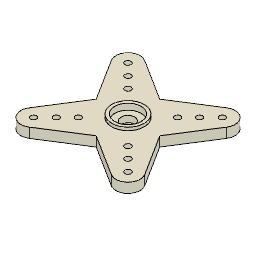
Square Servo Attachment (Autodesk Fusion 360 design; units mm, degrees)
Autodesk Fusion 360 part; units mm, degrees
sketch "Sketch1" plane through (0, 0, 0) normal (0, 1, 0) x (1, 0, 0)
  circle A0 centre (0, 0) radius 3.3909
  circle A1 centre (0, 0) radius 2.3368
  dimension "d1" = 6.7818
  dimension "d2" = 4.6736
  constraint coincident A0.centre A1.centre
  measures "d1" diameter of A0
  measures "d2" diameter of A1
extrude "Extrude1" add sketch "Sketch1" along normal blind 1.9304
sketch "Sketch2" plane through (0, 1.9304, 0) normal (0, 1, 0) x (-1, 0, 0)
  circle A0 centre (0, 0) radius 2.3368
  circle A1 centre (0, 0) radius 3.3909
  line L0 (-10.0076, 10.0076) -> (10.0076, 10.0076) construction
  line L1 (10.0076, 10.0076) -> (10.0076, -10.0076) construction
  line L2 (10.0076, -10.0076) -> (-10.0076, -10.0076) construction
  line L3 (-10.0076, -10.0076) -> (-10.0076, 10.0076) construction
  line L4 (-10.0076, 10.0076) -> (10.0076, -10.0076) construction
  line L5 (10.0076, 10.0076) -> (-10.0076, -10.0076) construction
  circle A2 centre (7.9709, -7.9709) radius 2.0367 construction
  circle A3 centre (-7.9709, -7.9709) radius 2.0367 construction
  circle A4 centre (-7.9709, 7.9709) radius 2.0367 construction
  circle A5 centre (7.9709, 7.9709) radius 2.0367 construction
  circle A6 centre (0, 0) radius 5.334 construction
  circle A7 centre (7.9709, -7.9709) radius 0.5
  circle A8 centre (-7.9709, -7.9709) radius 0.5
  circle A9 centre (7.9709, 7.9709) radius 0.5
  circle A10 centre (-7.9709, 7.9709) radius 0.5
  line L6 (8.4709, -7.9709) -> (-8.4709, -7.9709) construction
  line L7 (0, -5.334) -> (0, 5.334) construction
  line L8 (5.334, 0) -> (-5.334, 0) construction
  line L9 (9.4111, -6.5307) -> (6.5307, -9.4111) construction
  line L10 (-6.5307, -9.4111) -> (-9.4111, -6.5307) construction
  line L11 (-9.4111, 6.5307) -> (-6.5307, 9.4111) construction
  line L12 (9.4111, 6.5307) -> (6.5307, 9.4111) construction
  line L13 (5.334, 0) -> (9.6916, -6.8813)
  line L14 (5.334, 0) -> (9.6916, 6.8813)
  line L15 (0, 5.334) -> (6.8813, 9.6916)
  line L16 (0, 5.334) -> (-6.8813, 9.6916)
  line L17 (-5.334, 0) -> (-9.6916, 6.8813)
  line L18 (-5.334, 0) -> (-9.6916, -6.8813)
  line L19 (0, -5.334) -> (-6.8813, -9.6916)
  line L20 (0, -5.334) -> (6.8813, -9.6916)
  arc A11 (6.8813, -9.6916) -> (9.6916, -6.8813) centre (7.9709, -7.9709) ccw
  arc A12 (-9.6916, -6.8813) -> (-6.8813, -9.6916) centre (-7.9709, -7.9709) ccw
  arc A13 (-6.8813, 9.6916) -> (-9.6916, 6.8813) centre (-7.9709, 7.9709) ccw
  arc A14 (9.6916, 6.8813) -> (6.8813, 9.6916) centre (7.9709, 7.9709) ccw
  circle A15 centre (0, 0) radius 1.143
  dimension "d5" = 20.0152
  dimension "d6" = 20.0152
  dimension "d7" = 10.668
  dimension "d8" = 1
  dimension "d9" = 16.9418
  dimension "d10" = 2.286
  constraint horizontal L0
  constraint perpendicular L0 L1
  constraint parallel L0 L2
  constraint parallel L1 L3
  constraint coincident L4 A0.centre
  constraint coincident L5 A0.centre
  constraint coincident A0.centre A1.centre
  constraint coincident L4 A2.centre
  constraint coincident L5 A3.centre
  constraint coincident L4 A4.centre
  constraint coincident L5 A5.centre
  constraint tangent L2 A2
  constraint tangent L2 A3
  constraint tangent L3 A4
  constraint tangent L0 A5
  constraint equal A2 A3
  constraint equal A2 A4
  constraint equal A2 A5
  constraint concentric A2 A7
  constraint concentric A3 A8
  constraint concentric A5 A9
  constraint concentric A4 A10
  constraint equal A7 A8
  constraint equal A7 A9
  constraint equal A7 A10
  constraint coincident A7 L6.start
  constraint coincident A8 L6.end
  constraint coincident A2.centre L6
  constraint coincident A3.centre L6
  constraint coincident A6 L7.start
  constraint coincident A6 L7.end
  constraint coincident A0.centre L7
  constraint vertical L7
  constraint coincident A6 L8.start
  constraint coincident A6 L8.end
  constraint coincident A0.centre L8
  constraint horizontal L8
  constraint coincident A2 L9.start
  constraint coincident A2 L9.end
  constraint coincident A3 L10.start
  constraint coincident A3 L10.end
  constraint coincident A4 L11.start
  constraint coincident A4 L11.end
  constraint coincident A5 L12.start
  constraint coincident A5 L12.end
  constraint perpendicular L11 L12
  constraint coincident A2.centre L9
  constraint coincident A3.centre L10
  constraint coincident A4.centre L11
  constraint coincident A5.centre L12
  constraint perpendicular L4 L9
  constraint perpendicular L5 L10
  constraint perpendicular L4 L11
  constraint coincident A2 L13.end
  constraint coincident A5 L14.end
  constraint tangent A5 L14
  constraint coincident A5 L15.end
  constraint tangent A5 L15
  constraint coincident A4 L16.end
  constraint coincident A4 L17.end
  constraint tangent A4 L17
  constraint coincident A3 L18.end
  constraint coincident A3 L19.end
  constraint tangent A3 L19
  constraint coincident A2 L20.end
  constraint tangent A2 L13
  constraint tangent A2 L20
  constraint tangent A3 L18
  constraint tangent A4 L16
  constraint tangent L20 A11
  constraint tangent L18 A12
  constraint tangent L16 A13
  constraint tangent L15 A14
  measures "d5" distance of L1.end L2.end
  measures "d6" distance of L0.end L1.end
  measures "d7" diameter of A6
  measures "d8" diameter of A7
  measures "d9" distance of L6.start L6.end
  measures "d10" diameter of A15
extrude "Extrude2" add sketch "Sketch2" along normal blind 1.651 contours A0 | A1 | A7 | A8 | A9 | A10 | L13 L14 L15 L16 L17 L18 L19 L20 A11 A12 A13 A14
sketch "Sketch3" plane through (0, 3.5814, 0) normal (0, 1, 0) x (-1, 0, 0)
  circle A0 centre (0, 0) radius 1.143
  line L0 (5.334, 0) -> (9.6916, 6.8813)
  arc A1 (9.6916, 6.8813) -> (6.8813, 9.6916) centre (7.9709, 7.9709) ccw
  line L1 (6.8813, 9.6916) -> (0, 5.334)
  line L2 (0, 5.334) -> (-6.8813, 9.6916)
  arc A2 (-6.8813, 9.6916) -> (-9.6916, 6.8813) centre (-7.9709, 7.9709) ccw
  line L3 (-9.6916, 6.8813) -> (-5.334, 0)
  line L4 (-5.334, 0) -> (-9.6916, -6.8813)
  arc A3 (-9.6916, -6.8813) -> (-6.8813, -9.6916) centre (-7.9709, -7.9709) ccw
  line L5 (-6.8813, -9.6916) -> (0, -5.334)
  line L6 (0, -5.334) -> (6.8813, -9.6916)
  arc A4 (6.8813, -9.6916) -> (9.6916, -6.8813) centre (7.9709, -7.9709) ccw
  line L7 (9.6916, -6.8813) -> (5.334, 0)
  line L8 (-10.0076, 10.0076) -> (10.0076, 10.0076) construction
  line L9 (10.0076, 10.0076) -> (10.0076, -10.0076) construction
  line L10 (10.0076, -10.0076) -> (-10.0076, -10.0076) construction
  line L11 (-10.0076, -10.0076) -> (-10.0076, 10.0076) construction
  line L12 (-10.0076, 10.0076) -> (10.0076, -10.0076) construction
  line L13 (10.0076, 10.0076) -> (-10.0076, -10.0076) construction
  line L14 (8.2888, -8.2888) -> (-8.2888, 8.2888) construction
  line L15 (-8.2888, -8.2888) -> (8.2888, 8.2888) construction
  line L16 (-8.4455, 8.4455) -> (8.4455, 8.4455) construction
  line L17 (8.4455, 8.4455) -> (8.4455, -8.4455) construction
  line L18 (8.4455, -8.4455) -> (-8.4455, -8.4455) construction
  line L19 (-8.4455, -8.4455) -> (-8.4455, 8.4455) construction
  line L20 (-8.4455, 8.4455) -> (8.4455, -8.4455) construction
  line L21 (8.4455, 8.4455) -> (-8.4455, -8.4455) construction
  circle A5 centre (7.9104, -7.9104) radius 0.5351
  circle A6 centre (-7.9104, -7.9104) radius 0.5351
  circle A7 centre (-7.9104, 7.9104) radius 0.5351
  circle A8 centre (7.9104, 7.9104) radius 0.5351
  line L22 (-6.376, 6.376) -> (6.376, 6.376) construction
  line L23 (6.376, 6.376) -> (6.376, -6.376) construction
  line L24 (6.376, -6.376) -> (-6.376, -6.376) construction
  line L25 (-6.376, -6.376) -> (-6.376, 6.376) construction
  line L26 (-6.376, 6.376) -> (6.376, -6.376) construction
  line L27 (6.376, 6.376) -> (-6.376, -6.376) construction
  line L28 (-6.5278, 6.5278) -> (6.5278, 6.5278) construction
  line L29 (6.5278, 6.5278) -> (6.5278, -6.5278) construction
  line L30 (6.5278, -6.5278) -> (-6.5278, -6.5278) construction
  line L31 (-6.5278, -6.5278) -> (-6.5278, 6.5278) construction
  line L32 (-6.5278, 6.5278) -> (6.5278, -6.5278) construction
  line L33 (6.5278, 6.5278) -> (-6.5278, -6.5278) construction
  circle A9 centre (6.0095, -6.0095) radius 0.5183
  circle A10 centre (-6.0095, -6.0095) radius 0.5183
  circle A11 centre (-6.0095, 6.0095) radius 0.5183
  circle A12 centre (6.0095, 6.0095) radius 0.5183
  line L34 (-4.826, -4.826) -> (4.826, -4.826) construction
  line L35 (4.826, -4.826) -> (4.826, 4.826) construction
  line L36 (4.826, 4.826) -> (-4.826, 4.826) construction
  line L37 (-4.826, 4.826) -> (-4.826, -4.826) construction
  line L38 (-4.826, -4.826) -> (4.826, 4.826) construction
  line L39 (4.826, -4.826) -> (-4.826, 4.826) construction
  line L40 (-4.6338, -4.6338) -> (4.6338, -4.6338) construction
  line L41 (4.6338, -4.6338) -> (4.6338, 4.6338) construction
  line L42 (4.6338, 4.6338) -> (-4.6338, 4.6338) construction
  line L43 (-4.6338, 4.6338) -> (-4.6338, -4.6338) construction
  line L44 (-4.6338, -4.6338) -> (4.6338, 4.6338) construction
  line L45 (4.6338, -4.6338) -> (-4.6338, 4.6338) construction
  circle A13 centre (4.1698, -4.1698) radius 0.6562
  circle A14 centre (-4.1698, -4.1698) radius 0.6562
  circle A15 centre (-4.1698, 4.1698) radius 0.6562
  circle A16 centre (4.1698, 4.1698) radius 0.6562
  dimension "d13" = 23.4442
  dimension "d14" = 16.891
  dimension "d15" = 16.891
  dimension "d16" = 18.034
  dimension "d17" = 13.0556
  dimension "d18" = 13.1064
  dimension "d19" = 9.652
  constraint horizontal L8
  constraint perpendicular L8 L9
  constraint parallel L8 L10
  constraint parallel L9 L11
  constraint coincident L12 A0.centre
  constraint coincident L13 A0.centre
  constraint coincident A0.centre origin
  constraint tangent A4 L10
  constraint tangent A4 L9
  constraint coincident L12 L14.start
  constraint coincident L12 L14.end
  constraint midpoint A0.centre L14
  constraint coincident L13 L15.start
  constraint coincident L13 L15.end
  constraint midpoint A0.centre L15
  constraint equal L14 L15
  constraint horizontal L16
  constraint perpendicular L16 L17
  constraint parallel L16 L18
  constraint parallel L17 L19
  constraint coincident L20 A0.centre
  constraint coincident L21 A0.centre
  constraint coincident L12 A5.centre
  constraint coincident L15 A6.centre
  constraint coincident L14 A7.centre
  constraint coincident L21 A8.centre
  constraint coincident L14.start A5
  constraint coincident L15.start A6
  constraint coincident L14.end A7
  constraint coincident L15.end A8
  constraint tangent L18 A5
  constraint tangent L19 A6
  constraint tangent L19 A7
  constraint tangent L17 A8
  constraint horizontal L22
  constraint perpendicular L22 L23
  constraint parallel L22 L24
  constraint parallel L23 L25
  constraint coincident L26 A0.centre
  constraint coincident L27 A0.centre
  constraint coincident L20 L22.start
  constraint horizontal L28
  constraint perpendicular L28 L29
  constraint parallel L28 L30
  constraint parallel L29 L31
  constraint coincident L32 A0.centre
  constraint coincident L33 A0.centre
  constraint coincident L20 L28.start
  constraint coincident L14 A9.centre
  constraint coincident L33 A10.centre
  constraint coincident L32 A11.centre
  constraint coincident L33 A12.centre
  constraint coincident L23.end A9
  constraint coincident L24.end A10
  constraint coincident L22.start A11
  constraint coincident L22.end A12
  constraint tangent L30 A9
  constraint tangent L30 A10
  constraint tangent L28 A11
  constraint tangent L28 A12
  constraint horizontal L34
  constraint perpendicular L34 L35
  constraint parallel L34 L36
  constraint parallel L35 L37
  constraint coincident L38 A0.centre
  constraint coincident L39 A0.centre
  constraint coincident L15 L34.start
  constraint horizontal L40
  constraint perpendicular L40 L41
  constraint parallel L40 L42
  constraint parallel L41 L43
  constraint coincident L44 A0.centre
  constraint coincident L45 A0.centre
  constraint coincident L21 L40.start
  constraint coincident L39 A13.centre
  constraint coincident L13 A14.centre
  constraint coincident L26 A15.centre
  constraint coincident L15 A16.centre
  constraint coincident L40.end A13
  constraint coincident L40.start A14
  constraint coincident L42.end A15
  constraint coincident L41.end A16
  constraint tangent L34 A13
  constraint tangent L37 A14
  constraint tangent L37 A15
  constraint tangent L36 A16
  measures "d13" distance of L14.start L14.end
  measures "d14" distance of L17.end L18.end
  measures "d15" distance of L16.end L17.end
  measures "d16" distance of L22.start L23.end
  measures "d17" distance of L29.end L30.end
  measures "d18" distance of L40.end L42.end
  measures "d19" distance of L34.start L34.end
hole "Hole1" at (-7.9104, 3.5814, -7.9104) at (-6.0095, 3.5814, -6.0095) at (-4.1698, 3.5814, -4.1698) at (-7.9104, 3.5814, 7.9104) at (-6.0095, 3.5814, 6.0095) at (-4.1698, 3.5814, 4.1698) at (7.9104, 3.5814, 7.9104) at (6.0095, 3.5814, 6.0095) at (4.1698, 3.5814, 4.1698) at (7.9104, 3.5814, -7.9104) at (6.0095, 3.5814, -6.0095) at (4.1698, 3.5814, -4.1698) direction (0, -1, 0) diameter 1 end through all
sketch "Sketch4" plane through (0, 3.5814, 0) normal (0, 1, 0) x (-1, 0, 0)
  circle A0 centre (-6.0095, -6.0095) radius 0.5
  circle A1 centre (-4.1698, 4.1698) radius 0.5
  circle A2 centre (-7.9104, 7.9104) radius 0.5
  circle A3 centre (6.0095, 6.0095) radius 0.5
  circle A4 centre (4.1698, -4.1698) radius 0.5
  circle A5 centre (7.9104, -7.9104) radius 0.5
  circle A6 centre (6.0095, -6.0095) radius 0.5
  circle A7 centre (7.9104, 7.9104) radius 0.5
  circle A8 centre (4.1698, 4.1698) radius 0.5
  circle A9 centre (-6.0095, 6.0095) radius 0.5
  circle A10 centre (-7.9104, -7.9104) radius 0.5
  circle A11 centre (-4.1698, -4.1698) radius 0.5
  circle A12 centre (0, 0) radius 1.143
  line L0 (5.334, 0) -> (9.6916, 6.8813)
  arc A13 (9.6916, 6.8813) -> (6.8813, 9.6916) centre (7.9709, 7.9709) ccw
  line L1 (6.8813, 9.6916) -> (0, 5.334)
  line L2 (0, 5.334) -> (-6.8813, 9.6916)
  arc A14 (-6.8813, 9.6916) -> (-9.6916, 6.8813) centre (-7.9709, 7.9709) ccw
  line L3 (-9.6916, 6.8813) -> (-5.334, 0)
  line L4 (-5.334, 0) -> (-9.6916, -6.8813)
  arc A15 (-9.6916, -6.8813) -> (-6.8813, -9.6916) centre (-7.9709, -7.9709) ccw
  line L5 (-6.8813, -9.6916) -> (0, -5.334)
  line L6 (0, -5.334) -> (6.8813, -9.6916)
  arc A16 (6.8813, -9.6916) -> (9.6916, -6.8813) centre (7.9709, -7.9709) ccw
  line L7 (9.6916, -6.8813) -> (5.334, 0)
  circle A17 centre (0, 0) radius 2.7305
  circle A18 centre (0, 0) radius 2.2098
  dimension "d22" = 5.461
  dimension "d23" = 4.4196
  constraint coincident A12.centre A17.centre
  constraint concentric A12 A18
  measures "d22" diameter of A17
  measures "d23" diameter of A18
extrude "Extrude3" add sketch "Sketch4" along normal blind 0.508 contours A17
extrude "Extrude4" cut 1 faces at (-1.8417, 3.5814, -0.1666) along direction (0, -1, 0) blind 1.016 from surface at -0.508
extrude "Extrude5" cut 1 faces at (1.9259, 1.9304, 0.1729) along direction (0, 1, 0) blind 2.0066 from surface at -1.9304
